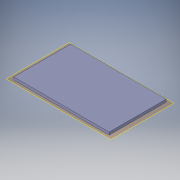
# Autodesk Inventor part: stamp5x3_empty
Saved by Autodesk Inventor 2019 (Build 230136000, 136)
## iProperties
Created: 2019-02-19
Part Number: stamp5x3_empty
Material: PET Plastic
Document SubType Name: Modeling
Designer: jmc
Density: 1.541 g/cm^3
Appearance: Slate Blue
Author: jmc
Autodesk Inventor part; units mm, degrees
ref_plane "YZ Plane" through (0, 0, 0) normal (1, 0, 0) x (0, 1, 0)
ref_plane "XZ Plane" through (0, 0, 0) normal (0, 1, 0) x (-1, 0, 0)
ref_plane "XY Plane" through (0, 0, 0) normal (0, 0, 1) x (1, 0, 0)
sketch "Sketch1" plane through (0, 0, 0) normal (0, 1, 0) x (-1, 0, 0)
  line L0 (24.925, 14.925) -> (-24.925, 14.925)
  line L1 (-24.925, 14.925) -> (-24.925, -14.925)
  line L2 (-24.925, -14.925) -> (24.925, -14.925)
  line L3 (24.925, 14.925) -> (-24.925, -14.925) construction
  line L4 (-24.925, 14.925) -> (24.925, -14.925) construction
  line L5 (24.925, -14.925) -> (24.925, 14.925)
  line L6 (24.925, 5) -> (24.925, 14.925)
  point P0 (0, 0)
  dimension "d0" = 49.85
  dimension "d1" = 29.85
  constraints: 14 end point, 3 parallel, 2 midpoint, 1 horizontal, 1 perpendicular
  measures "d0" distance of L2.end L1.end
  measures "d1" distance of L1.end L0.end
extrude "Extrusion1" add sketch "Sketch1" along normal blind 1.4
sketch "Sketch2" plane through (0, 0, 0) normal (0, -1, 0) x (1, 0, 0)
  point P0 (0, 0)
sketch "Sketch3" plane through (-24.925, 0, -14.925) normal (-1, 0, 0) x (0, 0, 1)
  point P0 (14.925, 0)
ref_plane "Work Plane1" through (0, 0, 0) normal (0, 1, 0) x (-1, 0, 0)
sketch "Sketch5" plane through (0, 0, 0) normal (0, 1, 0) x (-1, 0, 0)
  line L0 (-24.925, 14.925) -> (24.925, 14.925) projected
  line L1 (24.925, -14.925) -> (-24.925, -14.925) projected
  line L2 (24.925, 14.925) -> (24.925, -14.925) projected
  line L3 (-19.3821, 7.7039) -> (19.3821, 7.7039) construction
  line L4 (19.3821, 7.7039) -> (19.3821, -7.7039) construction
  line L5 (19.3821, -7.7039) -> (-19.3821, -7.7039) construction
  line L6 (-19.3821, -7.7039) -> (-19.3821, 7.7039) construction
  line L7 (-24.925, -14.925) -> (-24.925, 14.925) projected
  line L8 (-12.5833, 1.3105) -> (-16.2231, 1.3105)
  line L9 (-16.2231, 1.3105) -> (-16.2231, 3.7476)
  spline S0 degree 2 poles (-16.2231, 3.7476) (-16.2231, 4.8026) (-16.4552, 5.3301) (-16.8561, 5.3301) knots 0 0 0 1 2 2 2
  spline S1 degree 2 poles (-16.8561, 5.3301) (-17.3097, 5.3301) (-17.5524, 4.6866) (-17.5524, 3.6316) knots 0 0 0 1 2 2 2
  line L10 (-17.5524, 3.6316) -> (-17.5524, -2.8673)
  spline S2 degree 2 poles (-17.5524, -2.8673) (-17.5524, -3.8907) (-17.3097, -4.5131) (-16.8877, -4.5131) knots 0 0 0 1 2 2 2
  spline S3 degree 2 poles (-16.8877, -4.5131) (-16.4763, -4.5131) (-16.2231, -3.8907) (-16.2231, -2.7407) knots 0 0 0 1 2 2 2
  line L11 (-16.2231, -2.7407) -> (-16.2231, -0.9788)
  line L12 (-16.2231, -0.9788) -> (-12.5833, -0.9788)
  line L13 (-12.5833, -0.9788) -> (-12.5833, -1.5274)
  spline S4 degree 2 poles (-12.5833, -1.5274) (-12.5833, -3.7008) (-13.1952, -5.5154) (-15.3052, -6.8869) (-16.835, -6.8869) knots 0 0 0 1 2 3 3 3
  spline S5 degree 2 poles (-16.835, -6.8869) (-18.4386, -6.8869) (-20.517, -5.7264) (-21.1922, -3.6797) (-21.1922, -1.6224) knots 0 0 0 1 2 3 3 3
  line L14 (-21.1922, -1.6224) -> (-21.1922, 2.4711)
  spline S6 degree 2 poles (-21.1922, 2.4711) (-21.1922, 3.9797) (-20.9812, 5.4989) (-19.9578, 6.9021) (-18.1326, 7.7039) (-16.9405, 7.7039) knots 0 0 0 1 2 3 4 4 4
  spline S7 degree 2 poles (-16.9405, 7.7039) (-15.3369, 7.7039) (-13.2374, 6.459) (-12.5833, 4.6022) (-12.5833, 2.6399) knots 0 0 0 1 2 3 3 3
  line L15 (-12.5833, 2.6399) -> (-12.5833, 1.3105)
  line L16 (-11.2751, 7.4085) -> (-8.7008, 7.4085)
  spline S8 degree 2 poles (-8.7008, 7.4085) (-6.1266, 7.4085) (-4.3014, 7.0076) (-3.1515, 5.3723) (-3.1515, 3.5894) knots 0 0 0 1 2 3 3 3
  spline S9 degree 2 poles (-3.1515, 3.5894) (-3.1515, 1.9541) (-3.9638, 0.8252) (-5.156, 0.7092) knots 0 0 0 1 2 2 2
  spline S10 degree 2 poles (-5.156, 0.7092) (-4.0799, 0.4454) (-3.3308, -0.4513) (-3.1515, -1.2004) (-3.1515, -2.899) knots 0 0 0 1 2 3 3 3
  line L17 (-3.1515, -2.899) -> (-3.1515, -6.5915)
  line L18 (-3.1515, -6.5915) -> (-6.5381, -6.5915)
  line L19 (-6.5381, -6.5915) -> (-6.5381, -1.9389)
  spline S11 degree 2 poles (-6.5381, -1.9389) (-6.5381, -0.8206) (-6.8862, -0.2825) (-7.6353, -0.2825) knots 0 0 0 1 2 2 2
  line L20 (-7.6353, -0.2825) -> (-7.6353, -6.5915)
  line L21 (-7.6353, -6.5915) -> (-11.2751, -6.5915)
  line L22 (-11.2751, -6.5915) -> (-11.2751, 7.4085)
  line L23 (-7.6353, 5.0136) -> (-7.6353, 1.9013)
  spline S12 degree 2 poles (-7.6353, 1.9013) (-7.0234, 1.9013) (-6.5381, 2.239) (-6.5381, 3.1674) knots 0 0 0 1 2 2 2
  line L24 (-6.5381, 3.1674) -> (-6.5381, 3.9375)
  spline S13 degree 2 poles (-6.5381, 3.9375) (-6.5381, 4.6022) (-7.0128, 5.0136) (-7.6353, 5.0136) knots 0 0 0 1 2 2 2
  line L25 (4.5501, 7.4085) -> (6.639, -6.5915)
  line L26 (6.639, -6.5915) -> (2.9043, -6.5915)
  line L27 (2.9043, -6.5915) -> (2.7144, -4.07)
  line L28 (2.7144, -4.07) -> (1.4167, -4.07)
  line L29 (1.4167, -4.07) -> (1.2057, -6.5915)
  line L30 (1.2057, -6.5915) -> (-2.5712, -6.5915)
  line L31 (-2.5712, -6.5915) -> (-0.725, 7.4085)
  line L32 (-0.725, 7.4085) -> (4.5501, 7.4085)
  spline S14 degree 2 poles (2.6194, -1.5907) (2.3557, 0.783) (2.0708, 4.2857) knots 0 0 0 1 1 1
  spline S15 degree 2 poles (2.0708, 4.2857) (1.5222, 0.2661) (1.3745, -1.5907) knots 0 0 0 1 1 1
  line L33 (1.3745, -1.5907) -> (2.6194, -1.5907)
  line L34 (7.2615, 7.4085) -> (10.9329, 7.4085)
  spline S16 degree 2 poles (10.9329, 7.4085) (12.4205, 7.4085) (14.0241, 6.9443) (14.8259, 6.0581) (15.1108, 4.8026) (15.1108, 3.4944) knots 0 0 0 1 2 3 4 4 4
  line L35 (15.1108, 3.4944) -> (15.1108, 2.2706)
  spline S17 degree 2 poles (15.1108, 2.2706) (15.1108, 0.9307) (14.5516, -0.3036) (13.0746, -0.9577) (11.8824, -0.9577) knots 0 0 0 1 2 3 3 3
  line L36 (11.8824, -0.9577) -> (10.9013, -0.9577)
  line L37 (10.9013, -0.9577) -> (10.9013, -6.5915)
  line L38 (10.9013, -6.5915) -> (7.2615, -6.5915)
  line L39 (7.2615, -6.5915) -> (7.2615, 7.4085)
  line L40 (10.9013, 5.0136) -> (10.9013, 1.4477)
  spline S18 degree 2 poles (10.9013, 1.4477) (11.0595, 1.4371) (11.165, 1.4371) knots 0 0 0 1 1 1
  spline S19 degree 2 poles (11.165, 1.4371) (11.6714, 1.4371) (12.0618, 1.933) (12.0618, 2.7137) knots 0 0 0 1 2 2 2
  line L41 (12.0618, 2.7137) -> (12.0618, 3.8637)
  spline S20 degree 2 poles (12.0618, 3.8637) (12.0618, 4.5811) (11.6081, 5.0136) (10.9013, 5.0136) knots 0 0 0 1 2 2 2
  line L42 (19.6704, 7.4085) -> (19.4094, -2.7341)
  line L43 (19.4094, -2.7341) -> (17.8551, -2.7341)
  line L44 (17.8551, -2.7341) -> (17.5715, 7.4085)
  line L45 (17.5715, 7.4085) -> (19.6704, 7.4085)
  line L46 (19.5796, -6.5915) -> (17.6623, -6.5915)
  line L47 (17.6623, -6.5915) -> (17.6623, -4.6061)
  line L48 (17.6623, -4.6061) -> (19.5796, -4.6061)
  line L49 (19.5796, -4.6061) -> (19.5796, -6.5915)
  point P0 (0, 0)
  dimension "d13" = 29.85
  dimension "d14" = 49.85
  dimension "d16" = 38.7641
  dimension "d17" = 15.4078
  dimension "d18" = 7.2211
  dimension "d22" = 5.5429
  constraints: 2 other
  measures "d13" distance between parallel lines of L1 L0
  measures "d14" distance of L0.start L0.end
  measures "d16" distance of L3.start L3.end
  measures "d17" distance of L3.end L4.end
  measures "d18" distance between parallel lines of L0 L3
  measures "d22" distance between parallel lines of L7 L6
extrude "Extrusion4" add sketch "Sketch5" against normal blind 0.4 contours L8 L9 S0 S1 L10 S2 S3 L11 L12 L13 S4 S5 L14 S6 S7 L15 | L16 S8 S9 S10 L17 L18 L19 S11 L20 L21 L22 | L25 L26 L27 L28 L29 L30 L31 L32 | L34 S16 L35 S17 L36 L37 L38 L39 | L42 L43 L44 L45 | L46 L47 L48 L49
sketch "Sketch6" plane through (0, 0, 0) normal (0, -1, 0) x (1, 0, 0)
  line L0 (-24.925, 14.925) -> (-24.925, -14.925) projected
  line L1 (24.925, 14.925) -> (-24.925, 14.925) projected
  line L2 (24.925, -14.925) -> (24.925, 14.925) projected
  line L3 (-24.925, -14.925) -> (24.925, -14.925) projected
  line L4 (-22.925, 10.925) -> (-22.925, -10.925)
  line L5 (-20.925, -12.925) -> (20.925, -12.925)
  line L6 (22.925, -10.925) -> (22.925, 10.925)
  line L7 (20.925, 12.925) -> (-20.925, 12.925)
  arc A0 (-20.925, 12.925) -> (-22.925, 10.925) centre (-20.925, 10.925) ccw
  arc A1 (-22.925, -10.925) -> (-20.925, -12.925) centre (-20.925, -10.925) ccw
  arc A2 (20.925, -12.925) -> (22.925, -10.925) centre (20.925, -10.925) ccw
  arc A3 (22.925, 10.925) -> (20.925, 12.925) centre (20.925, 10.925) ccw
  line L8 (-20.925, 12.525) -> (20.925, 12.525)
  arc A4 (22.525, 10.925) -> (20.925, 12.525) centre (20.925, 10.925) ccw
  line L9 (22.525, 10.925) -> (22.525, -10.925)
  arc A5 (20.925, -12.525) -> (22.525, -10.925) centre (20.925, -10.925) ccw
  line L10 (20.925, -12.525) -> (-20.925, -12.525)
  arc A6 (-22.525, -10.925) -> (-20.925, -12.525) centre (-20.925, -10.925) ccw
  line L11 (-22.525, -10.925) -> (-22.525, 10.925)
  arc A7 (-20.925, 12.525) -> (-22.525, 10.925) centre (-20.925, 10.925) ccw
  point P0 (0, 0)
  dimension "d23" = 2
  dimension "d24" = 2
  dimension "d25" = 0.4
  constraints: 16 end point, 16 point on circle, 8 centre point, 8 tangent, 3 equal radius, 10 other
  measures "d23" distance between parallel lines of L1 L7
  measures "d24" radius of A0
  measures "d25" distance between parallel lines of L7 L8
extrude "Extrusion5" add sketch "Sketch6" along normal blind 0.4 contours A0 L7 A3 L6 A2 L5 A1 L4
equation "\"d18\" = 0.5 * d13 - 0.5 * d17"
equation "\"d22\" = 0.5 * d14 - 0.5 * d16"
body "Solid1"
